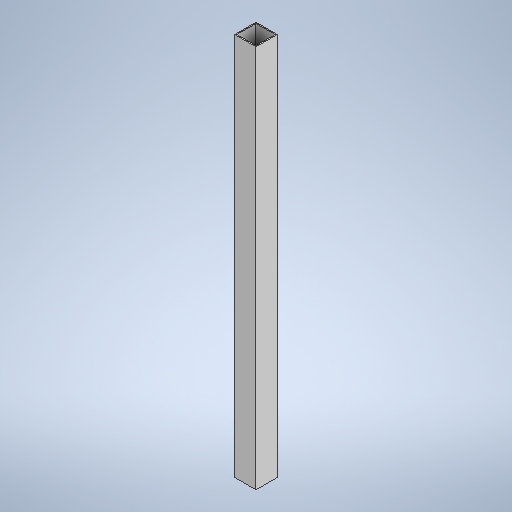
# Autodesk Inventor part: metalonmeio
Saved by Autodesk Inventor 2025 (Build 290162010, 162A)
## iProperties
Created: 2024-11-28
Part Number: metalonmeio
Material: Generic
Document SubType Name: Modeling
Designer: Bryan Ss
Density: 1 g/cm^3
Appearance: Default
Author: Bryan Ss
Autodesk Inventor part; units mm, degrees
ref_plane "YZ Plane" through (0, 0, 0) normal (1, 0, 0) x (0, 1, 0)
ref_plane "XZ Plane" through (0, 0, 0) normal (0, 1, 0) x (-1, 0, 0)
ref_plane "XY Plane" through (0, 0, 0) normal (0, 0, 1) x (1, 0, 0)
sketch "Sketch1" plane through (0, 0, 0) normal (0, 1, 0) x (-1, 0, 0)
  line L0 (0, 0) -> (50, 0)
  line L1 (50, 0) -> (50, -50)
  line L2 (50, -50) -> (0, -50)
  line L3 (0, -50) -> (0, 0)
  dimension "d0" = 50
  dimension "d1" = 50
  constraints: 8 end point, 2 parallel, 1 horizontal, 1 perpendicular
  measures "d0" distance of L1.end L2.end
  measures "d1" distance of L0.end L1.end
extrude "Extrusion1" add sketch "Sketch1" along normal blind 900
sketch "Sketch2" plane through (0, 900, 0) normal (0, 1, 0) x (1, 0, 0)
  line L0 (0, 50) -> (-50, 50) projected
  line L1 (-50, 50) -> (-50, 0) projected
  line L2 (-50, 0) -> (0, 0) projected
  line L3 (0, 0) -> (0, 50) projected
  line L4 (-47.5, 2.5) -> (-2.5, 2.5)
  line L5 (-2.5, 2.5) -> (-2.5, 47.5)
  line L6 (-2.5, 47.5) -> (-47.5, 47.5)
  line L7 (-47.5, 47.5) -> (-47.5, 2.5)
  line L8 (-47.5, 2.5) -> (-2.5, 47.5) construction
  line L9 (-2.5, 2.5) -> (-47.5, 47.5) construction
  point P0 (-25, 25)
  dimension "d4" = 45
  dimension "d5" = 45
  constraints: 12 end point, 2 midpoint, 2 parallel, 1 horizontal, 1 perpendicular
  measures "d4" distance of L6.end L5.end
  measures "d5" distance of L5.end L4.end
extrude "Extrusion2" cut sketch "Sketch2" against normal up to surface (900 mm away) contours L7 L6 L5 L4
body "Solid1"
